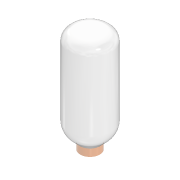
# Autodesk Inventor part: Бутылка_2
Saved by Autodesk Inventor 2022 (Build 260153000, 153)
## iProperties
Created: 2025-01-27
Part Number: Бутылка_2
Material: Типовые
Document SubType Name: Modeling
Designer: Ivan
Density: 1 g/cm^3
Appearance: Поликарбонат — прозрачный
Author: Ivan
Autodesk Inventor part; units mm, degrees
ref_plane "YZ Plane" through (0, 0, 0) normal (1, 0, 0) x (0, 1, 0)
ref_plane "XZ Plane" through (0, 0, 0) normal (0, 1, 0) x (-1, 0, 0)
ref_plane "XY Plane" through (0, 0, 0) normal (0, 0, 1) x (1, 0, 0)
sketch "Эскиз1" plane through (0, 0, 0) normal (0, 0, 1) x (1, 0, 0)
  line L0 (0, 0) -> (0, 59.8323)
  line L1 (0, 0) -> (17.5, 0)
  line L2 (17.5, 0) -> (17.5, 13)
  line L3 (17.5, 13) -> (28.7132, 24.2132)
  line L4 (37.5, 45.4264) -> (37.5, 168)
  line L5 (22.5, 183) -> (0, 183)
  line L6 (0, 183) -> (0, 0)
  arc A0 (37.5, 168) -> (22.5, 183) centre (22.5, 168) ccw
  arc A1 (28.7132, 24.2132) -> (37.5, 45.4264) centre (7.5, 45.4264) ccw
  point P0 (37.5, 33)
  dimension "d0" = 13
  dimension "d1" = 35
  dimension "d2" = 75
  dimension "d3" = 45
  dimension "d4" = 15
  dimension "d5" = 150
  dimension "d6" = 30
  constraints: 14 end point, 4 point on circle, 4 tangent, 3 perpendicular, 2 centre point, 2 point on line, 1 horizontal, 1 parallel, 1 vertical
  measures "d0" distance of L1.end L2.end
  measures "d1" diameter of L2 L0
  measures "d2" diameter of L4 L0
  measures "d3" angle of L4 L3
  measures "d4" radius of A0
  measures "d5" distance from line of point (37.5, 33) L5
  measures "d6" radius of A1
revolve "Вращение1" add sketch "Эскиз1" angle 360 about axis through (0, 0, 0) along (0, 1, 0)
